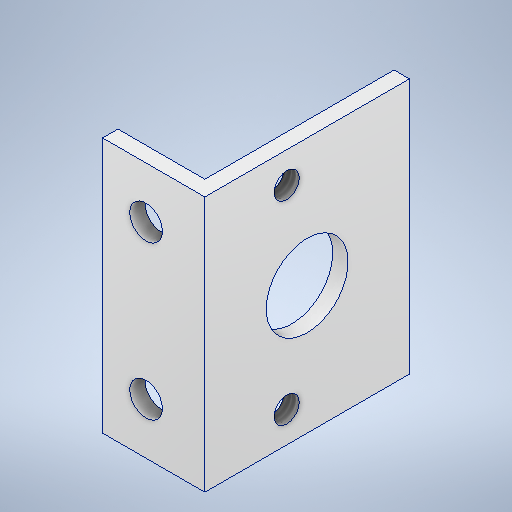
# Autodesk Inventor part: bearing_holder
Saved by Autodesk Inventor 2025 (Build 290162000, 162)
## iProperties
Created: 2024-04-25
Part Number: bearing_holder
Material: Hliník 6061
Document SubType Name: Modeling
Designer: rader
Density: 2.7 g/cm^3
Appearance: Hliník – plochý
Author: rader
Autodesk Inventor part; units mm, degrees
ref_plane "YZ Plane" through (0, 0, 0) normal (1, 0, 0) x (0, 1, 0)
ref_plane "XZ Plane" through (0, 0, 0) normal (0, 1, 0) x (-1, 0, 0)
ref_plane "XY Plane" through (0, 0, 0) normal (0, 0, 1) x (1, 0, 0)
sketch "Náčrt1" plane through (0, 0, 0) normal (0, 0, 1) x (1, 0, 0)
  line L0 (-10, 0) -> (0, 0)
  line L1 (0, 0) -> (0, 20)
  line L2 (0, 20) -> (-1.5, 20)
  line L3 (-1.5, 20) -> (-1.5, 1.5)
  line L4 (-1.5, 1.5) -> (-10, 1.5)
  line L5 (-10, 1.5) -> (-10, 0)
  line L6 (-12, 0) -> (2, 0) projected
  line L7 (0, 24) -> (0, -4) projected
  point P0 (0, 0)
  dimension "d0" = 20
  dimension "d1" = 10
  dimension "d2" = 1.5
  dimension "d3" = 1.5
  constraints: 12 end point, 5 perpendicular, 3 collinear, 1 horizontal
  measures "d0" distance of L0.end L1.end
  measures "d1" distance of L0.start L0.end
  measures "d2" distance between parallel lines of L3 L1
  measures "d3" distance between parallel lines of L4 L0
extrude "Vysunutí1" add sketch "Náčrt1" along normal mid plane 25
sketch "Náčrt2" plane through (-10, 1.5, 12.5) normal (0, 1, 0) x (1, 0, 0)
  line L0 (0, 0) -> (0, 25) projected
  line L1 (8.5, 0) -> (0, 0) projected
  line L2 (8.5, 25) -> (8.5, 0) projected
  line L3 (0, 25) -> (8.5, 25) projected
  point P0 (10, 12.5)
  point P1 (4.25, 20)
  point P2 (4.25, 5)
  point P3 (4.25, 0)
  dimension "d6" = 4.25
  dimension "d7" = 4.25
  dimension "d56" = 15
  dimension "d57" = 5
  constraints: 1 midpoint
  measures "d6" distance from line of L0 point (4.25, 5)
  measures "d7" distance from line of L0 point (4.25, 20)
  measures "d56" distance of point (4.25, 20) point (4.25, 5)
  measures "d57" distance from line of point (4.25, 5) L1
hole "Díra1" at (-5.75, 1.5, -7.5) at (-5.75, 1.5, 7.5) direction (0, -1, 0) diameter 3.2 end through all
sketch "Náčrt7" plane through (0, 0, 12.5) normal (1, 0, 0) x (0, 0, -1)
  line L0 (25, 20) -> (0, 20) projected
  line L1 (0, 0) -> (0, 20) projected
  line L2 (25, 0) -> (0, 0) projected
  line L3 (25, 20) -> (25, 0) projected
  point P0 (12.5, 0)
  point P1 (12.5, 10)
  dimension "d58" = 12.5
  dimension "d59" = 10
  measures "d58" distance from line of L3 point (12.5, 10)
  measures "d59" distance from line of L0 point (12.5, 10)
hole "Díra5" at (0, 10, 0) direction (-1, 0, 0) diameter 8 end through all
sketch "Náčrt8" plane through (0, 0, 12.5) normal (1, 0, 0) x (0, 0, -1)
  circle A0 centre (12.5, 10) radius 4 projected
  line L0 (25, 20) -> (0, 20) projected
  line L1 (0, 0) -> (0, 20) projected
  line L2 (25, 0) -> (0, 0) projected
  line L3 (25, 20) -> (25, 0) projected
  point P0 (12.5, 0)
  point P1 (22, 8)
  point P2 (3, 8)
  dimension "d67" = 8
  dimension "d68" = 8
  dimension "d69" = 3
  dimension "d70" = 3
  measures "d67" distance from line of L2 point (22, 8)
  measures "d68" distance from line of point (3, 8) L2
  measures "d69" distance from line of L3 point (22, 8)
  measures "d70" distance from line of L1 point (3, 8)
hole "Díra6" at (0, 8, -9.5) at (0, 8, 9.5) direction (-1, 0, 0) diameter 2.459 end through all thread size "M3x0.5" class "6H" standard "ISO Metric profile"
